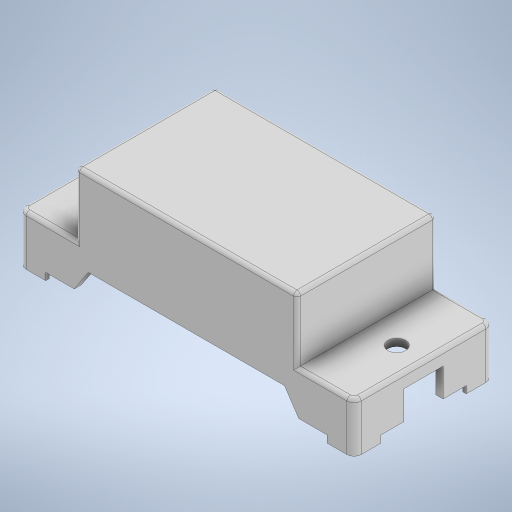
# Autodesk Inventor part: CO-1-01-12VoltFuseBox
Saved by Autodesk Inventor 2024 (Build 280153000, 153)
## iProperties
Created: 2024-01-24
Part Number: CO-1-01-12VoltFuseBox
Material: Generic
Document SubType Name: Modeling
Designer: ejned
Density: 1 g/cm^3
Appearance: Default
Author: ejned
Autodesk Inventor part; units mm, degrees
ref_plane "YZ Plane" through (0, 0, 0) normal (1, 0, 0) x (0, 1, 0)
ref_plane "XZ Plane" through (0, 0, 0) normal (0, 1, 0) x (-1, 0, 0)
ref_plane "XY Plane" through (0, 0, 0) normal (0, 0, 1) x (1, 0, 0)
sketch "Sketch1" plane through (0, 0, 0) normal (0, 1, 0) x (-1, 0, 0)
  line L0 (-59.69, 24.765) -> (59.69, 24.765)
  line L1 (59.69, 24.765) -> (59.69, -24.765)
  line L2 (59.69, -24.765) -> (-59.69, -24.765)
  line L3 (-59.69, -24.765) -> (-59.69, 24.765)
  point P0 (0, 0)
  dimension "d0" = 119.38
  dimension "d1" = 49.53
  dimension "d2" = 24.765
  dimension "d22" = 59.69
  constraints: 8 end point, 2 parallel, 1 horizontal, 1 perpendicular
  measures "d0" distance between parallel lines of L3 L1
  measures "d1" distance between parallel lines of L2 L0
  measures "d2" distance from line of point (0, 0) L0
  measures "d22" distance from line of point (0, 0) L1
extrude "Extrusion1" add sketch "Sketch1" along normal blind 40.64
sketch "Sketch2" plane through (0, 40.64, 0) normal (0, 1, 0) x (1, 0, 0)
  line L0 (-59.69, -24.765) -> (-39.37, -24.765)
  line L1 (-39.37, -24.765) -> (-39.37, 24.765)
  line L2 (-39.37, 24.765) -> (-59.69, 24.765)
  line L3 (-59.69, 24.765) -> (-59.69, -24.765)
  line L4 (59.69, -24.765) -> (59.69, 24.765) projected
  line L5 (59.69, -24.765) -> (39.37, -24.765)
  line L6 (39.37, -24.765) -> (39.37, 24.765)
  line L7 (39.37, 24.765) -> (59.69, 24.765)
  line L8 (59.69, 24.765) -> (59.69, -24.765)
  point P0 (0, 0)
  point P1 (59.69, 24.765)
  dimension "d6" = 20.32
  dimension "d7" = 20.32
  dimension "d8" = 49.53
  dimension "d9" = 49.53
  dimension "d10" = 78.74
  constraints: 16 end point, 4 parallel, 2 horizontal, 2 perpendicular, 1 point on line
  measures "d6" distance of L6.end L7.end
  measures "d7" distance of L1.end L2.end
  measures "d8" distance of L0.end L1.end
  measures "d9" distance of L5.end L6.end
  measures "d10" distance between parallel lines of L1 L6
extrude "Extrusion2" cut sketch "Sketch2" against normal blind 22.86
sketch "Sketch3" plane through (0, 0, 0) normal (0, -1, 0) x (1, 0, 0)
  circle A0 centre (50.165, 0) radius 3.175
  circle A1 centre (-50.165, 0) radius 3.175
  line L0 (-59.69, -24.765) -> (-59.69, 24.765) projected
  line L1 (59.69, 24.765) -> (59.69, -24.765) projected
  point P0 (0, 0)
  dimension "d13" = 6.35
  dimension "d14" = 6.35
  dimension "d15" = 6.35
  constraints: 2 centre point, 1 equal radius
  measures "d13" diameter of A0
  measures "d14" distance edge to line of A1 L0
  measures "d15" distance edge to line of A0 L1
extrude "Extrusion3" cut sketch "Sketch3" against normal blind 22.86
sketch "Sketch4" plane through (0, 0, 0) normal (0, -1, 0) x (1, 0, 0)
  line L0 (-57.15, -22.225) -> (57.15, -22.225)
  line L1 (57.15, -22.225) -> (57.15, 22.225)
  line L2 (57.15, 22.225) -> (-57.15, 22.225)
  line L3 (-57.15, 22.225) -> (-57.15, -22.225)
  line L4 (-59.69, -24.765) -> (-59.69, 24.765) projected
  line L5 (59.69, 24.765) -> (59.69, -24.765) projected
  line L6 (-59.69, 24.765) -> (59.69, 24.765) projected
  line L7 (59.69, -24.765) -> (-59.69, -24.765) projected
  point P0 (0, 0)
  dimension "d18" = 2.54
  dimension "d19" = 2.54
  dimension "d20" = 2.54
  dimension "d21" = 2.54
  constraints: 8 end point, 2 parallel, 1 horizontal, 1 perpendicular
  measures "d18" distance between parallel lines of L3 L4
  measures "d19" distance between parallel lines of L5 L1
  measures "d20" distance between parallel lines of L6 L2
  measures "d21" distance between parallel lines of L7 L0
extrude "Extrusion4" cut sketch "Sketch4" against normal blind 15.24 contours L3 L2 L1 L0
sketch "Sketch5" plane through (0, 15.24, 0) normal (0, -1, 0) x (1, 0, 0)
  line L0 (-57.15, 22.225) -> (57.15, 22.225) projected
  line L1 (-36.83, -22.225) -> (36.83, -22.225)
  line L2 (36.83, -22.225) -> (36.83, 22.225)
  line L3 (36.83, 22.225) -> (-36.83, 22.225)
  line L4 (-36.83, 22.225) -> (-36.83, -22.225)
  line L5 (-36.83, -22.225) -> (36.83, 22.225) construction
  line L6 (36.83, -22.225) -> (-36.83, 22.225) construction
  point P0 (0, 0)
  dimension "d25" = 73.66
  constraints: 12 end point, 2 midpoint, 2 parallel, 1 horizontal, 1 perpendicular, 1 point on line
  measures "d25" distance between parallel lines of L4 L2
extrude "Extrusion5" cut sketch "Sketch5" against normal blind 22.86
sketch "Sketch6" plane through (0, 0, 0) normal (0, -1, 0) x (1, 0, 0)
  line L0 (58.42, -23.495) -> (-58.42, 23.495) construction
  line L1 (-58.42, -23.495) -> (58.42, 23.495) construction
  line L2 (-59.69, -24.765) -> (-59.69, 24.765) projected
  line L3 (-59.69, 24.765) -> (59.69, 24.765) projected
  line L4 (50.165, 23.495) -> (50.165, 24.765)
  line L5 (-50.165, 23.495) -> (-50.165, 24.765)
  line L6 (-58.42, 15.24) -> (-59.69, 15.24)
  line L7 (-58.42, -15.24) -> (-59.69, -15.24)
  line L8 (-50.165, -23.495) -> (-50.165, -24.765)
  line L9 (50.165, -23.495) -> (50.165, -24.765)
  line L10 (59.69, -24.765) -> (-59.69, -24.765) projected
  line L11 (59.69, 24.765) -> (59.69, -24.765) projected
  line L12 (59.69, -15.24) -> (58.42, -15.24)
  line L13 (59.69, 15.24) -> (58.42, 15.24)
  line L14 (-50.165, 24.765) -> (50.165, 24.765)
  line L15 (59.69, -15.24) -> (59.69, 15.24)
  line L16 (50.165, -24.765) -> (-50.165, -24.765)
  line L17 (-59.69, -15.24) -> (-59.69, 15.24)
  line L18 (-57.15, -22.225) -> (-57.15, 22.225) projected
  line L19 (57.15, 22.225) -> (-57.15, 22.225)
  line L20 (-57.15, 22.225) -> (-57.15, -22.225)
  line L21 (-57.15, -22.225) -> (57.15, -22.225)
  line L22 (57.15, -22.225) -> (57.15, 22.225)
  line L23 (57.15, 22.225) -> (-57.15, -22.225) construction
  line L24 (-57.15, 22.225) -> (57.15, -22.225) construction
  line L25 (-58.42, -23.495) -> (-58.42, -15.24)
  line L26 (-58.42, 15.24) -> (-58.42, 23.495)
  line L27 (-58.42, 23.495) -> (-50.165, 23.495)
  line L28 (50.165, 23.495) -> (58.42, 23.495)
  line L29 (58.42, 23.495) -> (58.42, 15.24)
  line L30 (58.42, -15.24) -> (58.42, -23.495)
  line L31 (58.42, -23.495) -> (50.165, -23.495)
  line L32 (-50.165, -23.495) -> (-58.42, -23.495)
  point P0 (0, 0)
  point P1 (-59.055, 15.24)
  point P2 (-59.055, -15.24)
  dimension "d30" = 100.33
  dimension "d31" = 50.165
  dimension "d32" = 30.48
  dimension "d33" = 15.24
  dimension "d34" = 30.48
  dimension "d35" = 15.24
  dimension "d40" = 100.33
  dimension "d41" = 50.165
  constraints: 56 end point, 15 perpendicular, 14 parallel, 6 midpoint, 6 point on line, 3 collinear, 3 horizontal
  measures "d30" distance between parallel lines of L4 L5
  measures "d31" distance from line of point (0, 0) L5
  measures "d32" distance between parallel lines of L12 L13
  measures "d33" distance from line of point (0, 0) L13
  measures "d34" distance from line of L7 point (-59.055, 15.24)
  measures "d35" vertical distance of point (0, 0) point (-59.055, -15.24)
  measures "d40" distance of L9.end L8.end
  measures "d41" distance from line of point (0, 0) L8
extrude "Extrusion6" cut sketch "Sketch6" against normal blind 2.54 contours L2 L6 L26 L27 L5 L3 L4 L28 L29 L13 L11 L12 L30 L31 L9 L10 L8 L32 L25 L7 | L18 L19 L22 L21
sketch "Sketch7" plane through (0, 2.54, 0) normal (0, -1, 0) x (1, 0, 0)
  line L0 (-36.83, 22.225) -> (36.83, 22.225) projected
  line L1 (-39.37, 24.765) -> (39.37, 24.765) projected
  line L2 (34.925, 22.225) -> (-34.925, 22.225)
  line L3 (-34.925, 22.225) -> (-34.925, 24.765)
  line L4 (-34.925, 24.765) -> (34.925, 24.765)
  line L5 (34.925, 24.765) -> (34.925, 22.225)
  line L6 (50.165, -24.765) -> (-50.165, -24.765) projected
  line L7 (-57.15, -22.225) -> (57.15, -22.225) projected
  line L8 (-34.925, -24.765) -> (34.925, -24.765)
  line L9 (34.925, -24.765) -> (34.925, -22.225)
  line L10 (34.925, -22.225) -> (-34.925, -22.225)
  line L11 (-34.925, -22.225) -> (-34.925, -24.765)
  point P0 (0, 0)
  dimension "d42" = 69.85
  dimension "d43" = 34.925
  dimension "d44" = 69.85
  dimension "d45" = 34.925
  constraints: 16 end point, 4 parallel, 4 point on line, 2 horizontal, 2 perpendicular
  measures "d42" distance between parallel lines of L5 L3
  measures "d43" distance from line of point (0, 0) L3
  measures "d44" distance between parallel lines of L9 L11
  measures "d45" distance from line of point (0, 0) L11
extrude "Extrusion7" cut sketch "Sketch7" against normal blind 7.62
sketch "Sketch8" plane through (0, 2.54, 0) normal (0, -1, 0) x (1, 0, 0)
  line L0 (-57.15, 22.225) -> (-57.15, -22.225) projected
  line L1 (-59.69, -15.24) -> (-59.69, 15.24) projected
  line L2 (-57.15, -6.985) -> (-59.69, -6.985)
  line L3 (-59.69, -6.985) -> (-59.69, 6.985)
  line L4 (-59.69, 6.985) -> (-57.15, 6.985)
  line L5 (-57.15, 6.985) -> (-57.15, -6.985)
  point P0 (0, 0)
  dimension "d48" = 13.97
  dimension "d49" = 6.985
  constraints: 8 end point, 2 parallel, 2 point on line, 1 horizontal, 1 perpendicular
  measures "d48" distance between parallel lines of L2 L4
  measures "d49" distance from line of point (0, 0) L2
extrude "Extrusion8" cut sketch "Sketch8" against normal blind 10.16
mirror "Mirror1" about plane through (0, 0, 0) normal (1, 0, 0) of "Extrusion8"
fillet "Fillet1" radius 2.54 12 edges at (57.15, 8.89, 22.225) (58.42, 1.27, 23.495) (-58.42, 1.27, 23.495) (-57.15, 8.89, 22.225) (-58.42, 1.27, -23.495) (-57.15, 8.89, -22.225) (57.15, 8.89, -22.225) (58.42, 1.27, -23.495) (-59.69, 8.89, 24.765) (59.69, 8.89, 24.765) (-59.69, 8.89, -24.765) (59.69, 8.89, -24.765)
fillet "Fillet2" radius 1.27 18 edges at (-58.9461, 17.78, 24.0211) (-59.69, 17.78, 0) (-58.9461, 17.78, -24.0211) (-48.26, 17.78, -24.765) (-48.26, 17.78, 24.765) (58.9461, 17.78, 24.0211) (59.69, 17.78, 0) (58.9461, 17.78, -24.0211) (48.26, 17.78, -24.765) (48.26, 17.78, 24.765) (39.37, 29.21, 24.765) (0, 40.64, 24.765) (39.37, 40.64, 0) (39.37, 29.21, -24.765) (0, 40.64, -24.765) (-39.37, 40.64, 0) (-39.37, 29.21, 24.765) (-39.37, 29.21, -24.765)
chamfer "Chamfer1" distance 5.08 distance2 7.62 1 edges at (-34.925, 2.54, 23.495) measured on face at (-40.005, 2.54, 23.495)
chamfer "Chamfer2" distance 5.08 distance2 7.62 1 edges at (34.925, 2.54, 23.495) measured on face at (40.005, 2.54, 23.495)
chamfer "Chamfer3" distance 5.08 distance2 7.62 1 edges at (34.925, 2.54, -23.495) measured on face at (40.005, 2.54, -23.495)
chamfer "Chamfer4" distance 5.08 distance2 7.62 1 edges at (-34.925, 2.54, -23.495) measured on face at (-40.005, 2.54, -23.495)
body "Solid1"
